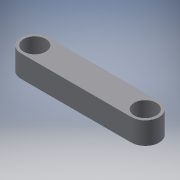
# Autodesk Inventor part: codo
Saved by Autodesk Inventor 2018 (Build 220112000, 112)
## iProperties
Created: 2021-07-10
Part Number: codo
Material: Genérico
Document SubType Name: Modeling
Designer: GABRIEL
Density: 1 g/cm^3
Appearance: Valor por defecto
Author: GABRIEL
Autodesk Inventor part; units mm, degrees
ref_plane "YZ Plane" through (0, 0, 0) normal (1, 0, 0) x (0, 1, 0)
ref_plane "XZ Plane" through (0, 0, 0) normal (0, 1, 0) x (-1, 0, 0)
ref_plane "XY Plane" through (0, 0, 0) normal (0, 0, 1) x (1, 0, 0)
sketch "Boceto1" plane through (0, 0, 0) normal (0, 0, 1) x (1, 0, 0)
  circle A0 centre (0, 0) radius 10
  circle A1 centre (100, 0) radius 10
  circle A2 centre (0, 0) radius 12.5
  circle A3 centre (100, 0) radius 12.5
  line L0 (0, 12.5) -> (100, 12.5)
  line L1 (0, -12.5) -> (100, -12.5)
  dimension "d0" = 20
  dimension "d1" = 20
  dimension "d2" = 25
  dimension "d3" = 25
  dimension "d4" = 100
  constraints: 4 centre point, 4 end point, 4 point on circle, 3 coincident, 2 tangent, 1 horizontal, 1 parallel
  measures "d0" diameter of A0
  measures "d1" diameter of A1
  measures "d2" diameter of A2
  measures "d3" diameter of A3
  measures "d4" distance of A1.centre point (0, 0)
extrude "Extrusión1" add sketch "Boceto1" along normal blind 30
